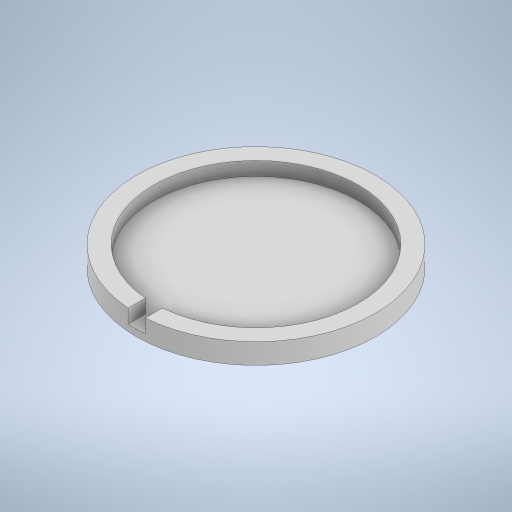
# Autodesk Inventor part: gps_case
Saved by Autodesk Inventor 2023 (Build 270158000, 158)
## iProperties
Created: 2024-02-08
Part Number: gps_case
Material: 일반
Document SubType Name: Modeling
Designer: ps737
Density: 1 g/cm^3
Appearance: 기본값
Author: ps737
Autodesk Inventor part; units mm, degrees
ref_plane "YZ Plane" through (0, 0, 0) normal (1, 0, 0) x (0, 1, 0)
ref_plane "XZ Plane" through (0, 0, 0) normal (0, 1, 0) x (-1, 0, 0)
ref_plane "XY Plane" through (0, 0, 0) normal (0, 0, 1) x (1, 0, 0)
sketch "스케치1" plane through (0, 0, 0) normal (0, 1, 0) x (-1, 0, 0)
  circle A0 centre (0, 0) radius 70
  circle A1 centre (0, 0) radius 60
  line L0 (-59.7913, -5) -> (-69.8212, -5)
  line L1 (-59.7913, 5) -> (-69.8212, 5)
  dimension "d0" = 140
  dimension "d1" = 120
  dimension "d7" = 5
  constraints: 4 end point, 4 point on circle, 2 centre point, 2 coincident, 2 horizontal
  measures "d0" diameter of A0
  measures "d1" diameter of A1
  measures "d7" distance from line of point (0, 0) L0
extrude "돌출1" add sketch "스케치1" along normal blind 12 contours A0 L0 A1 L1 | L1 A1 L0 A0
extrude "돌출2" add sketch "스케치1" along normal blind 4 contours A1
sketch "스케치2" plane through (0, 12, 0) normal (0, 1, 0) x (1, 0, 0)
  line L0 (5, -59.7913) -> (5, -69.8212)
  line L1 (-5, -59.7913) -> (-5, -69.8212)
  circle A0 centre (0, 0) radius 60 projected
  circle A1 centre (0, 0) radius 70 projected
  dimension "d8" = 10
  dimension "d9" = 5
  constraints: 4 end point, 4 point on circle, 2 vertical
  measures "d8" distance between parallel lines of L1 L0
  measures "d9" distance from line of point (0, 0) L0
extrude "돌출3" cut sketch "스케치2" against normal blind 8 contours L0 A1 L1 A0 picked at (3.8895, -63.1964)
